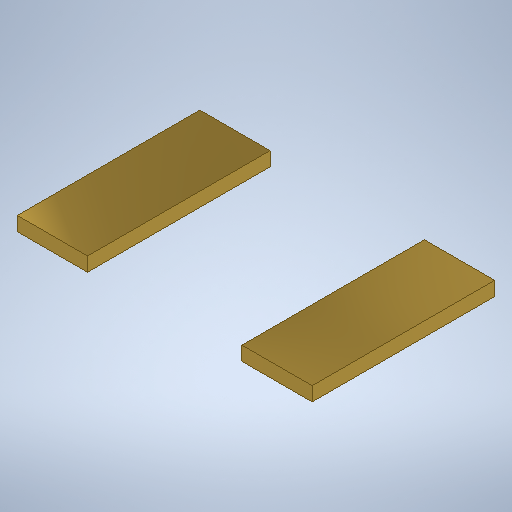
# Autodesk Inventor part: bottom_plates
Saved by Autodesk Inventor 2025 (Build 290162000, 162)
## iProperties
Created: 2025-09-09
Part Number: bottom_plates
Material: Gold
Document SubType Name: Modeling
Designer: jirne
Density: 19.3 g/cm^3
Appearance: Metal 1600F Hot
Author: jirne
Autodesk Inventor part; units mm, degrees
ref_plane "YZ Plane" through (0, 0, 0) normal (1, 0, 0) x (0, 1, 0)
ref_plane "XZ Plane" through (0, 0, 0) normal (0, 1, 0) x (-1, 0, 0)
ref_plane "XY Plane" through (0, 0, 0) normal (0, 0, 1) x (1, 0, 0)
sketch "Sketch1" plane through (0, 0, 0) normal (0, 0, 1) x (1, 0, 0)
  line L0 (0, 0) -> (1.27, 0)
  line L1 (1.27, 0) -> (1.27, 3.302)
  line L2 (1.27, 3.302) -> (0, 3.302)
  line L3 (0, 3.302) -> (0, 0)
  line L4 (4.064, 0) -> (5.334, 0)
  line L5 (5.334, 0) -> (5.334, 3.302)
  line L6 (5.334, 3.302) -> (4.064, 3.302)
  line L7 (4.064, 3.302) -> (4.064, 0)
  dimension "d0" = 1.27
  dimension "d1" = 3.302
  dimension "d2" = 1.27
  dimension "d3" = 3.302
  dimension "d4" = 5.334
  constraints: 16 end point, 4 parallel, 2 horizontal, 2 perpendicular, 1 collinear
  measures "d0" distance of L1.end L2.end
  measures "d1" distance of L0.end L1.end
  measures "d2" distance of L5.end L6.end
  measures "d3" distance of L4.end L5.end
  measures "d4" distance between parallel lines of L5 L3
extrude "Extrusion1" add sketch "Sketch1" along normal blind 0.254
body "Solid1"
